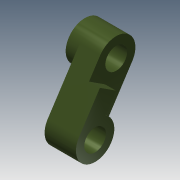
# Autodesk Inventor part: HbMiddle-RingCouplerLink01
Saved by Autodesk Inventor 2015 SP1 (Build 190203100, 203)
## iProperties
Created: 2015-02-23
Part Number: HbMiddle-RingCouplerLink01
Material: ナイロン 6/6
Document SubType Name: Modeling
Designer: Yamaura
Density: 1.13 g/cm^3
Appearance: 濃いオリーブ
Author: Yamaura
Autodesk Inventor part; units mm, degrees
ref_plane "YZ Plane" through (0, 0, 0) normal (1, 0, 0) x (0, 1, 0)
ref_plane "XZ Plane" through (0, 0, 0) normal (0, 1, 0) x (-1, 0, 0)
ref_plane "XY Plane" through (0, 0, 0) normal (0, 0, 1) x (1, 0, 0)
sketch "スケッチ1" plane through (0, 0, 0) normal (1, 0, 0) x (0, 1, 0)
  arc A0 (-2.5161, 1.6338) -> (2.5161, -1.6338) centre (0, 0) ccw
  circle A1 centre (5, 7.7) radius 1.7
  arc A2 (7.5161, 6.0662) -> (2.4839, 9.3338) centre (5, 7.7) ccw
  circle A3 centre (0, 0) radius 1.7
  line L0 (2.4839, 9.3338) -> (-2.5161, 1.6338)
  line L1 (7.5161, 6.0662) -> (2.5161, -1.6338)
  dimension "d1" = 3.4
  dimension "d2" = 6
  dimension "d3" = 3.4
  dimension "d4" = 5
  dimension "d5" = 7.7
  dimension "d8" = 3
  constraints: 4 centre point, 4 end point, 4 point on circle, 4 tangent, 3 coincident
  measures "d1" diameter of A1
  measures "d2" diameter of A2
  measures "d3" diameter of A3
  measures "d4" horizontal distance of A1.centre point (0, 0)
  measures "d5" vertical distance of A1.centre point (0, 0)
  measures "d8" radius of A0
extrude "押し出し1" add sketch "スケッチ1" against normal blind 6.6
sketch "スケッチ2" plane through (0, 0, 0) normal (1, 0, 0) x (0, 0, -1)
  circle A0 centre (0, 0) radius 1.7 projected
  circle A1 centre (-7.7, 5) radius 1.7 projected
  line L0 (-1.6338, -2.5161) -> (-9.3338, 2.4839) projected
  arc A2 (-1.6338, -2.5161) -> (1.6338, 2.5161) centre (0, 0) ccw projected
  line L1 (-6.0662, 7.5161) -> (1.6338, 2.5161) projected
  arc A3 (-6.0662, 7.5161) -> (-9.3338, 2.4839) centre (-7.7, 5) ccw projected
  circle A4 centre (0, 0) radius 3
  line L2 (-1.6338, -2.5161) -> (1.6338, 2.5161)
  dimension "d11" = 6
  constraints: 2 end point, 1 coincident, 1 midpoint, 1 perpendicular, 1 point on line, 3 other
extrude "押し出し2" cut sketch "スケッチ2" against normal blind 1.7 contours A4 L0 A3 L1
sketch "スケッチ3" plane through (-6.6, 0, 0) normal (-1, 0, 0) x (0, 0, 1)
  circle A0 centre (0, 0) radius 1.7 projected
  circle A1 centre (7.7, 5) radius 1.7 projected
  line L0 (1.6338, -2.5161) -> (9.3338, 2.4839) projected
  arc A2 (9.3338, 2.4839) -> (6.0662, 7.5161) centre (7.7, 5) ccw projected
  line L1 (6.0662, 7.5161) -> (-1.6338, 2.5161) projected
  arc A3 (-1.6338, 2.5161) -> (1.6338, -2.5161) centre (0, 0) ccw projected
  circle A4 centre (7.7, 5) radius 3
  line L2 (6.0662, 7.5161) -> (9.3338, 2.4839)
  line L3 (1.6338, -2.5161) -> (9.3338, 2.4839) projected
  dimension "d14" = 6
  constraints: 2 end point, 1 coincident, 1 midpoint, 1 perpendicular, 1 point on line, 3 other
extrude "押し出し3" cut sketch "スケッチ3" against normal blind 1.7 contours A4 L0 A3 L1
sketch "スケッチ5" plane through (-1.7, 0, 0) normal (1, 0, 0) x (0, 0, -1)
  arc A0 (-2.5161, 1.6338) -> (-1.6338, -2.5161) centre (0, 0) ccw
  line L0 (-1.6338, -2.5161) -> (-6.666, 0.7516)
  line L1 (-5.0322, 3.2676) -> (0, 0)
  line L2 (-6.666, 0.7516) -> (-5.0322, 3.2676)
  dimension "d18" = 6
  constraints: 6 end point, 2 point on circle, 1 centre point, 1 midpoint
  measures "d18" distance from line of L2 point (0, 0)
extrude "押し出し4" add sketch "スケッチ5" along normal up to surface (1.7 mm away)
